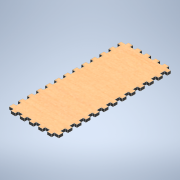
# Autodesk Inventor part: plate_bottom
Saved by Autodesk Inventor 2021 (Build 250183000, 183)
## iProperties
Created: 2021-03-07
Part Number: plate_bottom
Material: Generisch
Document SubType Name: Modeling
Designer: Tilman
Density: 1 g/cm^3
Appearance: Glänzend - Schwarz
Author: Tilman
Autodesk Inventor part; units mm, degrees
ref_plane "YZ Plane" through (0, 0, 0) normal (1, 0, 0) x (0, 1, 0)
ref_plane "XZ Plane" through (0, 0, 0) normal (0, 1, 0) x (-1, 0, 0)
ref_plane "XY Plane" through (0, 0, 0) normal (0, 0, 1) x (1, 0, 0)
sketch "Skizze1" plane through (0, 0, 0) normal (0, 1, 0) x (-1, 0, 0)
  line L0 (0, -3) -> (-5, -3)
  line L1 (-5, -3) -> (-5, 0)
  line L2 (-5, 0) -> (-10, 0)
  line L3 (-10, 0) -> (-10, -3)
  line L4 (-10, -3) -> (-15, -3)
  line L5 (-15, -3) -> (-15, 0)
  line L6 (-15, 0) -> (-20, 0)
  line L7 (-20, 0) -> (-20, -3)
  line L8 (-20, -3) -> (-25, -3)
  line L9 (-25, -3) -> (-25, 0)
  line L10 (-25, 0) -> (-30, 0)
  line L11 (-30, 0) -> (-30, -3)
  line L12 (-30, -3) -> (-35, -3)
  line L13 (-35, -3) -> (-35, 0)
  line L14 (-35, 0) -> (-40, 0)
  line L15 (-40, 0) -> (-40, -3)
  line L16 (-40, -3) -> (-45, -3)
  line L17 (-45, -3) -> (-45, 0)
  line L18 (-45, 0) -> (-50, 0)
  line L19 (-50, 0) -> (-50, -3)
  line L20 (-50, -3) -> (-55, -3)
  line L21 (-55, -3) -> (-55, -8)
  line L22 (-55, -8) -> (-52, -8)
  line L23 (-52, -8) -> (-52, -13)
  line L24 (-52, -13) -> (-55, -13)
  line L25 (-52, -18) -> (-52, -23)
  line L26 (-55, -13) -> (-55, -18)
  line L27 (-55, -18) -> (-52, -18)
  line L28 (-52, -23) -> (-55, -23)
  line L29 (-52, -28) -> (-52, -33)
  line L30 (-55, -23) -> (-55, -28)
  line L31 (-55, -28) -> (-52, -28)
  line L32 (-52, -33) -> (-55, -33)
  line L33 (-52, -38) -> (-52, -43)
  line L34 (-55, -33) -> (-55, -38)
  line L35 (-55, -38) -> (-52, -38)
  line L36 (-52, -43) -> (-55, -43)
  line L37 (-52, -48) -> (-52, -53)
  line L38 (-55, -43) -> (-55, -48)
  line L39 (-55, -48) -> (-52, -48)
  line L40 (-52, -53) -> (-55, -53)
  line L41 (-52, -58) -> (-52, -63)
  line L42 (-55, -53) -> (-55, -58)
  line L43 (-55, -58) -> (-52, -58)
  line L44 (-52, -63) -> (-55, -63)
  line L45 (-52, -68) -> (-52, -73)
  line L46 (-55, -63) -> (-55, -68)
  line L47 (-55, -68) -> (-52, -68)
  line L48 (-52, -73) -> (-55, -73)
  line L49 (-52, -78) -> (-52, -83)
  line L50 (-55, -73) -> (-55, -78)
  line L51 (-55, -78) -> (-52, -78)
  line L52 (-52, -83) -> (-55, -83)
  line L53 (-52, -88) -> (-52, -93)
  line L54 (-55, -83) -> (-55, -88)
  line L55 (-55, -88) -> (-52, -88)
  line L56 (-52, -93) -> (-55, -93)
  line L57 (-52, -98) -> (-52, -103)
  line L58 (-55, -93) -> (-55, -98)
  line L59 (-55, -98) -> (-52, -98)
  line L60 (-52, -103) -> (-55, -103)
  line L61 (-55, -127) -> (-50, -127)
  line L62 (-50, -127) -> (-50, -130)
  line L63 (-50, -130) -> (-45, -130)
  line L64 (-45, -130) -> (-45, -127)
  line L65 (-45, -127) -> (-40, -127)
  line L66 (-40, -130) -> (-35, -130)
  line L67 (-35, -130) -> (-35, -127)
  line L68 (-40, -127) -> (-40, -130)
  line L69 (-35, -127) -> (-30, -127)
  line L70 (-30, -130) -> (-25, -130)
  line L71 (-25, -130) -> (-25, -127)
  line L72 (-30, -127) -> (-30, -130)
  line L73 (-25, -127) -> (-20, -127)
  line L74 (-20, -130) -> (-15, -130)
  line L75 (-15, -130) -> (-15, -127)
  line L76 (-20, -127) -> (-20, -130)
  line L77 (-15, -127) -> (-10, -127)
  line L78 (-10, -130) -> (-5, -130)
  line L79 (-5, -130) -> (-5, -127)
  line L80 (-10, -127) -> (-10, -130)
  line L81 (-5, -127) -> (0, -127)
  line L82 (0, -123) -> (-3, -123)
  line L83 (-3, -123) -> (-3, -118)
  line L84 (-3, -118) -> (0, -118)
  line L85 (0, -118) -> (0, -113)
  line L86 (0, -108) -> (0, -103)
  line L87 (-3, -108) -> (0, -108)
  line L88 (-3, -113) -> (-3, -108)
  line L89 (0, -113) -> (-3, -113)
  line L90 (0, -98) -> (0, -93)
  line L91 (-3, -98) -> (0, -98)
  line L92 (-3, -103) -> (-3, -98)
  line L93 (0, -103) -> (-3, -103)
  line L94 (0, -88) -> (0, -83)
  line L95 (-3, -88) -> (0, -88)
  line L96 (-3, -93) -> (-3, -88)
  line L97 (0, -93) -> (-3, -93)
  line L98 (0, -78) -> (0, -73)
  line L99 (-3, -78) -> (0, -78)
  line L100 (-3, -83) -> (-3, -78)
  line L101 (0, -83) -> (-3, -83)
  line L102 (0, -68) -> (0, -63)
  line L103 (-3, -68) -> (0, -68)
  line L104 (-3, -73) -> (-3, -68)
  line L105 (0, -73) -> (-3, -73)
  line L106 (0, -58) -> (0, -53)
  line L107 (-3, -58) -> (0, -58)
  line L108 (-3, -63) -> (-3, -58)
  line L109 (0, -63) -> (-3, -63)
  line L110 (0, -48) -> (0, -43)
  line L111 (-3, -48) -> (0, -48)
  line L112 (-3, -53) -> (-3, -48)
  line L113 (0, -53) -> (-3, -53)
  line L114 (0, -38) -> (0, -33)
  line L115 (-3, -38) -> (0, -38)
  line L116 (-3, -43) -> (-3, -38)
  line L117 (0, -43) -> (-3, -43)
  line L118 (0, -28) -> (0, -23)
  line L119 (-3, -28) -> (0, -28)
  line L120 (-3, -33) -> (-3, -28)
  line L121 (0, -33) -> (-3, -33)
  line L122 (-52, -108) -> (-52, -113)
  line L123 (-55, -103) -> (-55, -108)
  line L124 (-55, -108) -> (-52, -108)
  line L125 (-52, -113) -> (-55, -113)
  line L126 (-52, -118) -> (-52, -123)
  line L127 (-55, -113) -> (-55, -118)
  line L128 (-55, -118) -> (-52, -118)
  line L129 (-52, -123) -> (-55, -123)
  line L130 (0, -18) -> (0, -13)
  line L131 (-3, -18) -> (0, -18)
  line L132 (-3, -23) -> (-3, -18)
  line L133 (0, -23) -> (-3, -23)
  line L134 (0, -8) -> (0, -3)
  line L135 (-3, -8) -> (0, -8)
  line L136 (-3, -13) -> (-3, -8)
  line L137 (0, -13) -> (-3, -13)
  line L138 (-55, -123) -> (-55, -127)
  line L139 (0, -127) -> (0, -123)
  point P0 (0, 0)
  dimension "d0" = 3
  dimension "d1" = 5
  dimension "d4" = 10
  dimension "d11" = 10
  dimension "d16" = 130
  dimension "d19" = 10
  dimension "d33" = 10
  constraints: 280 end point, 21 point on line, 17 equal length, 15 perpendicular, 8 horizontal, 5 vertical, 4 collinear, 2 horizontal alignment, 2 vertical alignment, 257 other
  measures "d0" distance of L0.end L1.end
  measures "d1" distance of L0.start L0.end
  measures "d4" distance of L2.end L6.end
  measures "d11" distance of L22.end L25.start
  measures "d16" distance of L18.end L62.end
  measures "d19" distance of L61.start L65.start
  measures "d33" distance of L84.end L86.start
extrude "Extrusion1" add sketch "Skizze1" along normal blind 3
